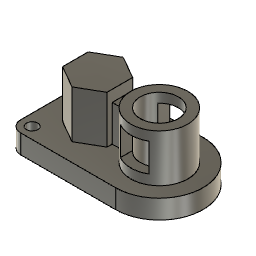
drawing_25 (Autodesk Fusion 360 design; units mm, degrees)
Autodesk Fusion 360 part; units mm, degrees
note: some values were not read from the file. Set by a fixed rule: which sketch regions a step uses.
sketch "Sketch1" plane through (0, 0, 0) normal (0, 0, 1) x (1, 0, 0)
  line L0 (-56, 46) -> (56, 46)
  line L1 (56, 46) -> (56, -46)
  line L2 (56, -46) -> (-56, -46)
  line L3 (-56, -46) -> (-56, 46)
  line L4 (-56, 46) -> (56, -46) construction
  line L5 (56, 46) -> (-56, -46) construction
  dimension "d1" = 92
  dimension "d2" = 112
  constraint horizontal L0
  constraint perpendicular L0 L1
  constraint parallel L0 L2
  constraint parallel L1 L3
  constraint coincident L4 origin
  constraint coincident L5 origin
  measures "d1" distance of L0.end L1.end
  measures "d2" distance of L0.start L0.end
extrude "Extrude1" add sketch "Sketch1" along normal blind 20
sketch "Sketch2" plane through (0, 0, 0) normal (0, 0, -1) x (1, 0, 0)
  line L0 (56, 46) -> (-56, 46)
  line L1 (-56, 46) -> (-56, -46)
  line L2 (-56, -46) -> (56, -46)
  line L3 (56, -46) -> (56, 46)
  circle A0 centre (56, 0) radius 46
  dimension "d5" = 92
  constraint midpoint L3 A0.centre
  measures "d5" diameter of A0
extrude "Extrude2" add sketch "Sketch2" against normal blind 20 contours L3 A0 picked at (67.5882, 10.0412)
sketch "Sketch3" plane through (0, 0, 20) normal (0, 0, 1) x (-1, 0, 0)
  line L0 (56, 46) -> (-56, 46)
  arc A0 (-56, 46) -> (-56, -46) centre (-56, 0) ccw
  line L1 (-56, -46) -> (56, -46)
  line L2 (56, -46) -> (56, 46)
  circle A1 centre (-56, 0) radius 30
  dimension "d8" = 60
  constraint concentric A0 A1
  measures "d8" diameter of A1
extrude "Extrude3" add sketch "Sketch3" along normal blind 50 contours A1
ref_plane "WorkPlane1" through (56, -30, 48.1933) normal (0, -1, 0) x (-1, 0, 0)
sketch "Sketch4" plane through (56, -30, 48.1933) normal (0, -1, 0) x (1, 0, 0)
  line L0 (30, 21.8067) -> (-30, 21.8067)
  line L1 (0, -48.1933) -> (46, -48.1933)
  line L2 (46, -28.1933) -> (30, -28.1933)
  line L3 (-112, -48.1933) -> (-112, -28.1933)
  line L4 (-112, -48.1933) -> (0, -48.1933)
  line L5 (-30, -28.1933) -> (-112, -28.1933)
  line L6 (30, -28.1933) -> (30, 21.8067)
  line L7 (-30, -28.1933) -> (-30, 21.8067)
  line L8 (46, -48.1933) -> (46, -28.1933)
  line L9 (0, 21.8067) -> (0, 11.8067) construction
  line L10 (0, 11.8067) -> (0, -3.1933) construction
  line L11 (15, 11.8067) -> (-15, 11.8067)
  line L12 (-15, 11.8067) -> (-15, -18.1933)
  line L13 (-15, -18.1933) -> (15, -18.1933)
  line L14 (15, -18.1933) -> (15, 11.8067)
  line L15 (15, 11.8067) -> (-15, -18.1933) construction
  line L16 (-15, 11.8067) -> (15, -18.1933) construction
  point P0 (0, -3.1933)
  dimension "d12" = 10
  dimension "d13" = 15
  dimension "d14" = 30
  dimension "d15" = 30
  constraint midpoint L0 L9.start
  constraint perpendicular L0 L9
  constraint perpendicular L0 L10
  constraint horizontal L11
  constraint perpendicular L11 L12
  constraint parallel L11 L13
  constraint parallel L12 L14
  constraint coincident L15 P0
  constraint coincident L16 P0
  constraint coincident P0 L10.end
  measures "d12" distance of L9.start L9.end
  measures "d13" distance of L9.end P0
  measures "d14" distance of L12.end L13.end
  measures "d15" distance of L11.end L12.end
extrude "Extrude4" cut sketch "Sketch4" against normal blind 100 contours L11 L12 L13 L14
sketch "Sketch5" plane through (0, 0, 70) normal (0, 0, 1) x (-1, 0, 0)
  circle A0 centre (-56, 0) radius 30
  circle A1 centre (-56, 0) radius 20
  dimension "d18" = 40
  constraint concentric A0 A1
  measures "d18" diameter of A1
extrude "Extrude5" cut sketch "Sketch5" against normal blind 120 contours A1
sketch "Sketch6" plane through (0, 0, 20) normal (0, 0, 1) x (-1, 0, 0)
  circle A0 centre (-56, 0) radius 30
  line L0 (56, 46) -> (-56, 46)
  arc A1 (-56, 46) -> (-56, -46) centre (-56, 0) ccw
  line L1 (-56, -46) -> (56, -46)
  line L2 (56, -46) -> (56, 46)
  line L3 (56, -46) -> (56, -34) construction
  line L4 (56, -34) -> (44, -34) construction
  circle A2 centre (44, -34) radius 12
  line L5 (56, 46) -> (56, 34) construction
  line L6 (56, 34) -> (44, 34) construction
  circle A3 centre (44, 34) radius 12
  circle A4 centre (44, 34) radius 6
  circle A5 centre (44, -34) radius 6
  dimension "d21" = 12
  dimension "d22" = 12
  dimension "d23" = 24
  dimension "d24" = 12
  dimension "d25" = 12
  dimension "d26" = 24
  dimension "d27" = 12
  dimension "d28" = 12
  constraint coincident L1.end L2.start
  constraint perpendicular L1 L3
  constraint perpendicular L2 L4
  constraint coincident L4.end A2.centre
  constraint coincident L0.start L2.end
  constraint perpendicular L0 L5
  constraint perpendicular L5 L6
  constraint coincident L6.end A3.centre
  constraint concentric A3 A4
  constraint concentric A2 A5
  measures "d21" distance of L1.end L3.end
  measures "d22" distance of L3.end L4.end
  measures "d23" diameter of A2
  measures "d24" distance of L0.start L5.end
  measures "d25" distance of L5.end L6.end
  measures "d26" diameter of A3
  measures "d27" diameter of A4
  measures "d28" diameter of A5
extrude "Extrude6" cut sketch "Sketch6" against normal blind 30 contours A4 | A5
sketch "Sketch7" plane through (0, 0, 20) normal (0, 0, 1) x (-1, 0, 0)
  circle A0 centre (44, -34) radius 6
  circle A1 centre (44, 34) radius 6
  circle A2 centre (-56, 0) radius 30
  line L0 (56, 46) -> (-56, 46)
  arc A3 (-56, 46) -> (-56, -46) centre (-56, 0) ccw
  line L1 (-56, -46) -> (56, -46)
  line L2 (56, -46) -> (56, 46)
  circle A4 centre (44, -34) radius 12
  circle A5 centre (44, 34) radius 12
  dimension "d31" = 24
  dimension "d32" = 24
  constraint concentric A0 A4
  constraint concentric A1 A5
  measures "d31" diameter of A4
  measures "d32" diameter of A5
extrude "Extrude7" cut sketch "Sketch7" against normal blind 40 contours L0 L2 A5 | L1 L2 A4
sketch "Sketch8" plane through (0, 0, 20) normal (0, 0, 1) x (-1, 0, 0)
  arc A0 (56, 34) -> (44, 46) centre (44, 34) ccw
  line L0 (44, 46) -> (-56, 46)
  arc A1 (-56, 46) -> (-56, -46) centre (-56, 0) ccw
  line L1 (-56, -46) -> (44, -46)
  arc A2 (44, -46) -> (56, -34) centre (44, -34) ccw
  line L2 (56, -34) -> (56, 34)
  circle A3 centre (44, -34) radius 6
  circle A4 centre (44, 34) radius 6
  circle A5 centre (-56, 0) radius 30
  line L3 (44, -34) -> (9, -34) construction
  line L4 (9, 34) -> (9, 0) construction
  line L5 (9, -27) -> (32.3827, -13.5)
  line L6 (32.3827, -13.5) -> (32.3827, 13.5)
  line L7 (32.3827, 13.5) -> (9, 27)
  line L8 (9, 27) -> (-14.3827, 13.5)
  line L9 (-14.3827, 13.5) -> (-14.3827, -13.5)
  line L10 (-14.3827, -13.5) -> (9, -27)
  line L11 (9, -34) -> (9, -27)
  arc A6 (-14.3827, -11.3688) -> (-12.537, -14.5656) centre (9, 0) ccw construction
  arc A7 (-12.537, 14.5656) -> (-14.3827, 11.3688) centre (9, 0) ccw construction
  arc A8 (10.8457, 25.9344) -> (7.1543, 25.9344) centre (9, 0) ccw construction
  arc A9 (10.8457, -25.9344) -> (32.3827, -11.3688) centre (9, 0) ccw construction
  arc A10 (32.3827, 11.3688) -> (30.537, 14.5656) centre (9, 0) ccw construction
  point P0 (9, 0)
  dimension "d35" = 35
  dimension "d36" = 52
  constraint coincident A2.centre A3.centre
  constraint horizontal L3
  constraint perpendicular L0 L4
  constraint coincident P0 L4.end
  constraint perpendicular L3 L11
  constraint coincident L5 A9.start
  constraint coincident L10 A6.end
  constraint coincident L9 A7.end
  constraint coincident L9 A6.start
  constraint concentric A6 A9
  constraint coincident L8 A8.end
  constraint coincident L8 A7.start
  constraint concentric A7 A9
  constraint coincident L7 A10.end
  constraint coincident L7 A8.start
  constraint concentric A8 A9
  constraint coincident L6 A9.end
  constraint coincident L6 A10.start
  constraint concentric A9 A10
  measures "d35" distance of A2.centre L3.end
  measures "d36" diameter of A9
extrude "Extrude8" add sketch "Sketch8" along normal blind 50 contours L5 L6 L7 L8 L9 L10
sketch "Sketch9" plane through (0, 0, 20) normal (0, 0, 1) x (-1, 0, 0)
  line L0 (-14.3827, -13.5) -> (-14.3827, 13.5)
  line L1 (-14.3827, 13.5) -> (9, 27)
  line L2 (9, 27) -> (32.3827, 13.5)
  line L3 (32.3827, 13.5) -> (32.3827, -13.5)
  line L4 (32.3827, -13.5) -> (9, -27)
  line L5 (9, -27) -> (-14.3827, -13.5)
  arc A0 (56, 34) -> (44, 46) centre (44, 34) ccw
  line L6 (44, 46) -> (-56, 46)
  arc A1 (-56, 46) -> (-56, -46) centre (-56, 0) ccw
  line L7 (-56, -46) -> (44, -46)
  arc A2 (44, -46) -> (56, -34) centre (44, -34) ccw
  line L8 (56, -34) -> (56, 34)
  circle A3 centre (44, -34) radius 6
  circle A4 centre (44, 34) radius 6
  circle A5 centre (-56, 0) radius 30
  line L9 (-14.3827, -13.5) -> (9, -27)
  line L10 (9, -27) -> (32.3827, -13.5)
  line L11 (32.3827, -13.5) -> (32.3827, 13.5)
  line L12 (32.3827, 13.5) -> (9, 27)
  line L13 (9, 27) -> (-14.3827, 13.5)
  line L14 (-14.3827, 13.5) -> (-14.3827, -13.5)
  circle A6 centre (-56, 0) radius 20
  circle A7 centre (-56, 0) radius 30
  line L15 (-10, 0) -> (-29.7237, 0) construction
  line L16 (-10, 0) -> (-10, -8) construction
  line L17 (-10, -8) -> (-32.4254, -8)
  line L18 (-32.4254, -8) -> (-32.4254, 8)
  line L19 (-32.4254, 8) -> (-10, 8)
  line L20 (-10, 8) -> (-10, -8)
  dimension "d39" = 8
  dimension "d40" = 16
  constraint perpendicular L0 L15
  constraint perpendicular L15 L16
  constraint horizontal L17
  constraint vertical L18
  constraint horizontal L19
  constraint vertical L20
  measures "d39" distance of L15.start L16.end
  measures "d40" distance of L16.end L19.end
extrude "Extrude9" add sketch "Sketch9" along normal blind 38 contours L0 A5 L14 A7 L17 L19 | L0 L14 L17 L19 L20 | A5 A7 L17 L18 L19 picked at (-30.2836, 0)
equation "d1 = 68 mm + 12 mm + 12 mm"
equation "d5 = 46 mm + 46 mm"
equation "d41 = 50 mm - 12 mm"
